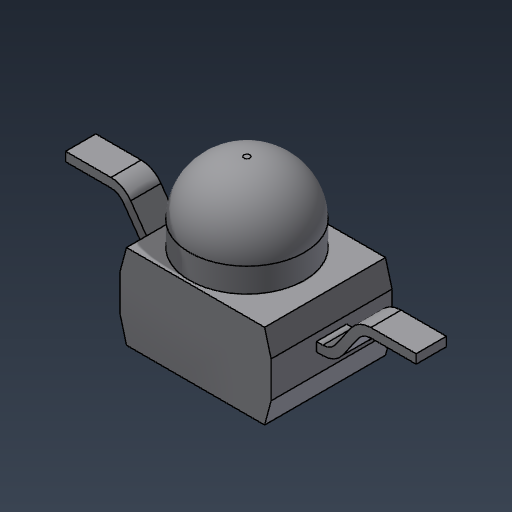
# Autodesk Inventor part: IR LED Reverse Gullwing
Saved by Autodesk Inventor 2023.1 (Build 271208000, 208)
## iProperties
Created: 2015-09-04
Part Number: IR LED Reverse Gullwing
Material: Allgemein
Document SubType Name: Modeling
Designer: rYan
Density: 1 g/cm^3
Appearance: Vorgabe
Mass: 0.00998671 g
Surface Area: 0.318102 cm^2
Volume: 0.00998671 cm^3
Author: rYan
Autodesk Inventor part; units mm, degrees
ref_plane "YZ Plane" through (0, 0, 0) normal (1, 0, 0) x (0, 1, 0)
ref_plane "XZ Plane" through (0, 0, 0) normal (0, 1, 0) x (-1, 0, 0)
ref_plane "XY Plane" through (0, 0, 0) normal (0, 0, 1) x (1, 0, 0)
sketch "Skizze1" plane through (0, 0, 0) normal (0, 0, 1) x (1, 0, 0)
  line L0 (-1.25, -1) -> (1.25, -1)
  line L1 (1.25, -1) -> (1.25, 1)
  line L2 (1.25, 1) -> (-1.25, 1)
  line L3 (-1.25, 1) -> (-1.25, -1)
  line L4 (-1.25, -1) -> (1.25, 1) construction
  line L5 (1.25, -1) -> (-1.25, 1) construction
  point P0 (0, 0)
  dimension "d0" = 2.5
  dimension "d1" = 2
  constraints: 12 end point, 2 midpoint, 2 parallel, 1 horizontal, 1 perpendicular
  measures "d0" distance of L2.end L1.end
  measures "d1" distance of L1.end L0.end
extrude "Extrusion1" add sketch "Skizze1" against normal blind 1.4
sketch "Skizze2" plane through (0, 0, 0) normal (0, 0, 1) x (1, 0, 0)
  line L0 (-1.25, -1) -> (1.25, -1) projected
  line L1 (1.25, -1) -> (1.25, 1) projected
  line L2 (1.25, 1) -> (-1.25, 1) projected
  line L3 (-1.25, 1) -> (-1.25, -1) projected
  circle A0 centre (-0.15, 0) radius 0.95
  line L4 (-1.75, 0) -> (1.75, 0) projected
  point P0 (0, 0)
  dimension "d4" = 1.9
  dimension "d5" = 1.1
  constraints: 1 centre point, 1 point on line
  measures "d4" diameter of A0
  measures "d5" distance from line of A0.centre L3
extrude "Extrusion2" add sketch "Skizze2" along normal blind 1.3 contours L4 A0 | A0 L4
fillet "Rundung1" radius 0.9 1 edges at (-1.1, 0, 1.3)
sketch "Skizze3" plane through (0, 0, 0) normal (0, 1, 0) x (-1, 0, 0)
  line L0 (1.25, 0) -> (-1.25, 0) projected
  line L1 (1.25, 0) -> (1.25, -1.4) projected
  line L2 (-1.25, -1.4) -> (1.25, -1.4) projected
  line L3 (-1.25, 0) -> (-1.25, -1.4) projected
  line L4 (1.25, 0) -> (1.25, -1.4) projected
  line L5 (1.25, -0.6) -> (1.3565, -0.6)
  arc A0 (1.3565, -0.6) -> (1.6227, -0.4614) centre (1.3565, -0.275) ccw
  line L6 (1.6227, -0.4614) -> (1.8838, -0.0886)
  arc A1 (2.15, 0.05) -> (1.8838, -0.0886) centre (2.15, -0.275) ccw
  line L7 (2.15, 0.05) -> (2.9, 0.05)
  line L8 (0, -1.94) -> (0, 1.84) projected
  line L9 (2.15, -0.275) -> (1.3565, -0.275) construction
  point P0 (0, 0)
  dimension "d9" = 55
  dimension "d10" = 2.9
  dimension "d11" = 2.15
  dimension "d12" = 0.05
  dimension "d13" = 0.6
  constraints: 8 end point, 4 point on circle, 4 tangent, 2 centre point, 1 equal radius, 1 horizontal, 1 parallel, 1 perpendicular, 1 point on line
  measures "d9" angle of L5 L6
  measures "d10" distance from line of L7.end L8
  measures "d11" distance from line of L8 L7.start
  measures "d12" distance between parallel lines of L0 L7
  measures "d13" distance between parallel lines of L0 L5
sketch "Skizze4" plane through (-1.25, -1, 0) normal (-1, 0, 0) x (0, 0, 1)
  line L0 (-0.675, 1.25) -> (-0.525, 1.25)
  line L1 (-0.525, 1.25) -> (-0.525, 0.75)
  line L2 (-0.525, 0.75) -> (-0.675, 0.75)
  line L3 (-0.675, 0.75) -> (-0.675, 1.25)
  line L4 (-0.675, 1.25) -> (-0.525, 0.75) construction
  line L5 (-0.525, 1.25) -> (-0.675, 0.75) construction
  point P0 (0, 1)
  point P1 (-0.6, 1)
  point P2 (-0.6, 1)
  point P3 (-0.6, 1)
  dimension "d14" = 0.15
  dimension "d15" = 0.5
  constraints: 12 end point, 2 midpoint, 2 parallel, 1 horizontal, 1 perpendicular
  measures "d14" distance of L1.end L2.end
  measures "d15" distance of L0.end L1.end
sweep "Sweeping1" add profiles "Skizze4" path "Skizze3" path curves L5 A0 L6 A1 L7
mirror "Spiegeln1" about plane through (0, 0, 0) normal (1, 0, 0) of "Sweeping1"
chamfer "Fase1" distance 0.4 angle 15 2 edges at (-1.25, 0, 0) (-1.25, 0, -1.4) measured on face at (-1.25, 0.0833, -1.1583)
chamfer "Fase2" distance 0.4 angle 15 2 edges at (1.25, 0, 0) (1.25, 0, -1.4) measured on face at (1.25, -0.0833, -1.1583)
